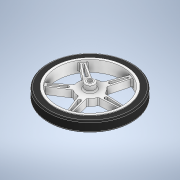
# Autodesk Inventor part: wheel
Saved by Autodesk Inventor 2021 (Build 250183000, 183)
## iProperties
Created: 2022-05-14
Part Number: wheel
Material: Generic
Document SubType Name: Modeling
Designer: ermoz
Density: 1 g/cm^3
Appearance: Default
Author: ermoz
Autodesk Inventor part; units mm, degrees
ref_plane "YZ Plane" through (0, 0, 0) normal (1, 0, 0) x (0, 1, 0)
ref_plane "XZ Plane" through (0, 0, 0) normal (0, 1, 0) x (-1, 0, 0)
ref_plane "XY Plane" through (0, 0, 0) normal (0, 0, 1) x (1, 0, 0)
sketch "Sketch1" plane through (0, 0, 0) normal (0, 1, 0) x (-1, 0, 0)
  circle A0 centre (0, 0) radius 30
  circle A1 centre (0, 0) radius 25.25
  dimension "d0" = 60
  dimension "d1" = 50.5
  constraints: 2 centre point, 2 coincident
  measures "d0" diameter of A0
  measures "d1" diameter of A1
extrude "Extrusion1" add sketch "Sketch1" along normal blind 7.5
sketch "Sketch2" plane through (0, 7.5, 0) normal (0, 1, 0) x (1, 0, 0)
  circle A0 centre (0, 0) radius 23.5
  circle A1 centre (0, 0) radius 25.25
  dimension "d4" = 47
  constraints: 2 centre point, 1 coincident
  measures "d4" diameter of A0
extrude "Extrusion2" add sketch "Sketch2" along normal blind 0.25 and the other way blind 7.75 separate body
fillet "Fillet1" radius 1 2 edges at (30, 7.5, 0) (30, 0, 0)
sketch "Sketch3" plane through (0, 7.75, 0) normal (0, 1, 0) x (1, 0, 0)
  circle A0 centre (0, 0) radius 8.5
  dimension "d10" = 17
  constraints: 1 centre point, 1 coincident
  measures "d10" diameter of A0
extrude "Extrusion3" add sketch "Sketch3" against normal blind 6.5 bodies 2
extrude "Extrusion4" cut sketch "Sketch3" against normal blind 1.5 bodies 2
sketch "Sketch4" plane through (0, 6.25, 0) normal (0, 1, 0) x (1, 0, 0)
  line L0 (5, 2.5) -> (23.8822, 1.5)
  line L1 (5, 2.5) -> (5, -2.5)
  line L2 (5, -2.5) -> (23.8822, -1.5)
  line L3 (23.8822, -1.5) -> (23.8822, 1.5)
  line L4 (0, 0) -> (1.9067, 0)
  line L5 (22.6235, 0.4453) -> (10.461, 1.0894)
  line L6 (10.461, 1.0894) -> (10.461, -1.0894)
  line L7 (10.461, -1.0894) -> (22.6235, -0.4453)
  line L8 (22.6235, -0.4453) -> (22.6235, 0.4453)
  line L9 (-0.8326, 5.5278) -> (5.9534, 23.1768)
  line L10 (-0.8326, 5.5278) -> (3.9227, 3.9827)
  line L11 (3.9227, 3.9827) -> (8.8066, 22.2498)
  line L12 (8.8066, 22.2498) -> (5.9534, 23.1768)
  line L13 (0, 0) -> (0.5892, 1.8134)
  line L14 (6.5676, 21.6538) -> (2.1965, 10.2856)
  line L15 (2.1965, 10.2856) -> (4.2687, 9.6123)
  line L16 (4.2687, 9.6123) -> (7.4145, 21.3786)
  line L17 (7.4145, 21.3786) -> (6.5676, 21.6538)
  line L18 (-5.5145, 0.9164) -> (-20.2027, 12.8241)
  line L19 (-5.5145, 0.9164) -> (-2.5756, 4.9615)
  line L20 (-2.5756, 4.9615) -> (-18.4394, 15.2511)
  line L21 (-18.4394, 15.2511) -> (-20.2027, 12.8241)
  line L22 (0, 0) -> (-1.5425, 1.1207)
  line L23 (-18.5645, 12.9375) -> (-9.1034, 5.2675)
  line L24 (-9.1034, 5.2675) -> (-7.8228, 7.0301)
  line L25 (-7.8228, 7.0301) -> (-18.041, 13.658)
  line L26 (-18.041, 13.658) -> (-18.5645, 12.9375)
  line L27 (-2.5756, -4.9615) -> (-18.4394, -15.2511)
  line L28 (-2.5756, -4.9615) -> (-5.5145, -0.9164)
  line L29 (-5.5145, -0.9164) -> (-20.2027, -12.8241)
  line L30 (-20.2027, -12.8241) -> (-18.4394, -15.2511)
  line L31 (0, 0) -> (-1.5425, -1.1207)
  line L32 (-18.041, -13.658) -> (-7.8228, -7.0301)
  line L33 (-7.8228, -7.0301) -> (-9.1034, -5.2675)
  line L34 (-9.1034, -5.2675) -> (-18.5645, -12.9375)
  line L35 (-18.5645, -12.9375) -> (-18.041, -13.658)
  line L36 (3.9227, -3.9827) -> (8.8066, -22.2498)
  line L37 (3.9227, -3.9827) -> (-0.8326, -5.5278)
  line L38 (-0.8326, -5.5278) -> (5.9534, -23.1768)
  line L39 (5.9534, -23.1768) -> (8.8066, -22.2498)
  line L40 (0, 0) -> (0.5892, -1.8134)
  line L41 (7.4145, -21.3786) -> (4.2687, -9.6123)
  line L42 (4.2687, -9.6123) -> (2.1965, -10.2856)
  line L43 (2.1965, -10.2856) -> (6.5676, -21.6538)
  line L44 (6.5676, -21.6538) -> (7.4145, -21.3786)
  dimension "d15" = 3
  dimension "d16" = 5
  dimension "d17" = 5
  dimension "d20" = 360
  constraints: 90 end point, 10 point on line, 3 parallel, 2 coincident, 2 vertical, 1 horizontal, 1 symmetric about line, 101 other
  measures "d15" distance of L2.end L0.end
  measures "d16" distance of L0.start L1.end
  measures "d17" distance from line of L1 L4.start
extrude "Extrusion5" add sketch "Sketch4" against normal up to surface (5 mm away) bodies 2
fillet "Fillet2" radius 1 20 edges at (4.2687, 3.75, -9.6123) (2.1965, 3.75, -10.2856) (-7.8228, 3.75, -7.0301) (-9.1034, 3.75, -5.2675) (-5.2421, 3.75, -6.691) (0.3081, 3.75, -8.4944) (-7.9835, 3.75, -2.9179) (-7.9835, 3.75, 2.9179) (-9.1034, 3.75, 5.2675) (-7.8228, 3.75, 7.0301) (-5.2421, 3.75, 6.691) (0.3081, 3.75, 8.4944) (2.1965, 3.75, 10.2856) (4.2687, 3.75, 9.6123) (4.7436, 3.75, 7.0532) (8.1739, 3.75, 2.3319) (10.461, 3.75, 1.0894) (10.461, 3.75, -1.0894) (8.1739, 3.75, -2.3319) (4.7436, 3.75, -7.0532)
fillet "Fillet3" radius 1 10 edges at (-19.8671, 3.75, -12.5519) (-18.0768, 3.75, -15.0159) (5.7983, 3.75, -22.7734) (8.695, 3.75, -21.8323) (23.4506, 3.75, -1.5229) (23.4506, 3.75, 1.5229) (5.7983, 3.75, 22.7734) (8.695, 3.75, 21.8323) (-19.8671, 3.75, 12.5519) (-18.0768, 3.75, 15.0159)
sketch "Sketch5" plane through (0, 6.25, 0) normal (0, 1, 0) x (1, 0, 0)
  circle A0 centre (0, 0) radius 3.25
  dimension "d26" = 6.5
  constraints: 1 centre point, 1 coincident
  measures "d26" diameter of A0
extrude "Extrusion6" add sketch "Sketch5" along normal blind 5 bodies 2
fillet "Fillet4" radius 1 2 edges at (-3.25, 6.25, 0) (-3.25, 11.25, 0)
sketch "Sketch6" plane through (0, 11.25, 0) normal (0, 1, 0) x (1, 0, 0)
  circle A0 centre (0, 0) radius 3.25 projected
  circle A1 centre (0, 0) radius 1.5
  dimension "d30" = 3
  constraints: 1 centre point, 1 coincident
  measures "d30" diameter of A1
extrude "Extrusion7" cut sketch "Sketch6" against normal through all contours A1 bodies 2
fillet "Fillet5" radius 0.5 10 edges at (6.5676, 3.75, 21.6538) (7.4145, 3.75, 21.3786) (22.6235, 3.75, -0.4453) (22.6235, 3.75, 0.4453) (6.5676, 3.75, -21.6538) (7.4145, 3.75, -21.3786) (-18.041, 3.75, -13.658) (-18.5645, 3.75, -12.9375) (-18.5645, 3.75, 12.9375) (-18.041, 3.75, 13.658)
body "Solid1"
body "Solid2"
